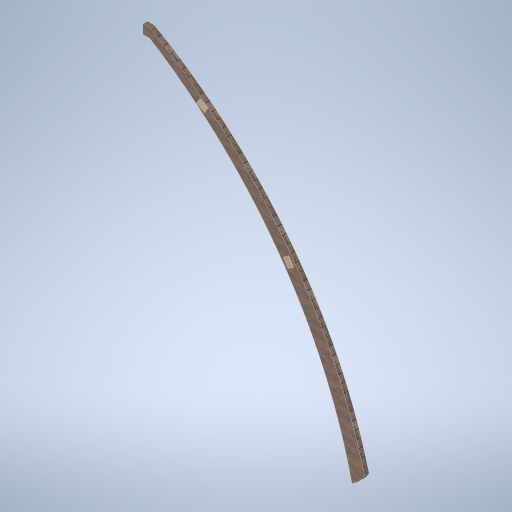
# Autodesk Inventor part: curve_beam_03
Saved by Autodesk Inventor 2024.2 (Build 282272000, 272)
## iProperties
Created: 2024-05-20
Part Number: curve_beam_03
Material: Wood (Maple)
Document SubType Name: Modeling
Designer: LOSTER_1
Density: 0.67 g/cm^3
Appearance: Natural Maple - Glossy Dark Tint
Author: LOSTER_1
Autodesk Inventor part; units mm, degrees
ref_plane "YZ Plane" through (0, 0, 0) normal (1, 0, 0) x (0, 1, 0)
ref_plane "XZ Plane" through (0, 0, 0) normal (0, 1, 0) x (-1, 0, 0)
ref_plane "XY Plane" through (0, 0, 0) normal (0, 0, 1) x (1, 0, 0)
sketch "Sketch1" plane through (0, 0, 0) normal (0, 0, 1) x (1, 0, 0)
  ellipse E0 centre (4015.7888, -1667.4861) end of major axis (4015.7888, -2467.4861) minor radius 800 (4424.4298, -2355.2452) -> (4701.6709, -2079.2696) ccw
  arc A0 (4701.6709, -2079.2696) -> (-25.36, 4106.1752) centre (-4980.6691, -4579.7278) ccw
  arc A1 (4424.4298, -2355.2452) -> (-25.36, 3906.647) centre (-5326.6573, -4572.5185) ccw
  arc A2 (4424.4298, -2355.2452) -> (4701.6709, -2079.2696) centre (4015.7888, -1667.4861) ccw
  line L0 (-25.36, 4106.1752) -> (-175.36, 4106.1752)
  line L1 (-175.36, 4106.1752) -> (-175.36, 3906.647)
  line L2 (-175.36, 3906.647) -> (-25.36, 3906.647)
  point P0 (0, 0)
  dimension "d0" = 10000
  dimension "d1" = 10000
  dimension "d2" = 150
  constraints: 6 end point, 6 point on circle, 3 centre point, 2 perpendicular, 1 horizontal, 4 other
  measures "d0" radius of A0
  measures "d1" radius of A1
  measures "d2" distance of L0.start L0.end
extrude "Extrusion1" add sketch "Sketch1" along normal blind 100
sketch "Sketch2" plane through (0, 0, 100) normal (0, 0, 1) x (1, 0, 0)
  line L0 (1082.7501, 3318.1208) -> (1255.9551, 3218.1208)
  line L1 (1255.9551, 3218.1208) -> (1180.9551, 3088.2169)
  line L2 (1180.9551, 3088.2169) -> (1007.7501, 3188.2169)
  line L3 (1007.7501, 3188.2169) -> (1082.7501, 3318.1208)
  line L4 (1082.7501, 3318.1208) -> (1180.9551, 3088.2169) construction
  line L5 (1255.9551, 3218.1208) -> (1007.7501, 3188.2169) construction
  line L6 (1082.7501, 3318.1208) -> (1282.7501, 3318.1208) construction
  line L7 (2908.3705, 1201.3295) -> (3023.0858, 1037.499)
  line L8 (3023.0858, 1037.499) -> (3145.9586, 1123.5355)
  line L9 (3145.9586, 1123.5355) -> (3031.2433, 1287.3659)
  line L10 (3031.2433, 1287.3659) -> (2908.3705, 1201.3295)
  line L11 (2908.3705, 1201.3295) -> (3145.9586, 1123.5355) construction
  line L12 (3023.0858, 1037.499) -> (3031.2433, 1287.3659) construction
  line L13 (2908.3705, 1201.3295) -> (3108.3705, 1201.3295) construction
  point P0 (0, 0)
  point P1 (1131.8526, 3203.1688)
  point P2 (3027.1645, 1162.4325)
  dimension "d5" = 200
  dimension "d6" = 30
  dimension "d7" = 150
  dimension "d8" = 200
  dimension "d9" = 55
  dimension "d10" = 150
  constraints: 28 end point, 4 midpoint, 4 parallel, 2 equal length, 2 horizontal, 2 perpendicular
  measures "d5" distance of L0.start L0.end
  measures "d6" angle of L0 L6
  measures "d7" distance of L0.end L1.end
  measures "d8" distance of L7.start L7.end
  measures "d9" angle of L7 L13
  measures "d10" distance of L8.end L7.end
extrude "Extrusion2" cut sketch "Sketch2" against normal through all
body "Solid1"
